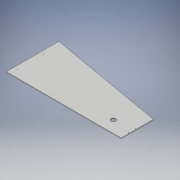
# Autodesk Inventor part: pinball-case-left-wall-outer
Saved by Autodesk Inventor 2017 (Build 210142000, 142)
## iProperties
Created: 2017-02-27
Part Number: pinball-case-left-wall-outer
Material: Generic
Document SubType Name: Modeling
Designer: John
Density: 1 g/cm^3
Appearance: Default
Author: John
Autodesk Inventor part; units mm, degrees
ref_plane "YZ Plane" through (0, 0, 0) normal (1, 0, 0) x (0, 1, 0)
ref_plane "XZ Plane" through (0, 0, 0) normal (0, 1, 0) x (-1, 0, 0)
ref_plane "XY Plane" through (0, 0, 0) normal (0, 0, 1) x (1, 0, 0)
sketch "Sketch1" plane through (0, 0, 0) normal (0, 1, 0) x (-1, 0, 0)
  line L0 (0, 0) -> (-590, 0)
  line L1 (-590, 0) -> (-590, -165.9671)
  line L2 (-590, -165.9671) -> (0, -165.9671)
  line L3 (0, -165.9671) -> (0, 0)
  line L4 (0, -165.9671) -> (0, -270)
  line L5 (0, -270) -> (-590, -165.9671)
  dimension "d0" = 590
  dimension "d28" = 270
  dimension "d29" = 10
  constraints: 12 end point, 2 parallel, 1 horizontal, 1 perpendicular, 1 vertical
  measures "d0" distance of L2.end L1.end
  measures "d28" distance of L0.start L4.end
  measures "d29" angle of L2 L5
extrude "Extrusion1" add sketch "Sketch1" along normal blind 3
sketch "Sketch3" plane through (0, 3, 0) normal (0, 1, 0) x (1, 0, 0)
  circle A0 centre (585.75, 41.75) radius 1.25
  circle A1 centre (585.75, 78.75) radius 1.25
  line L0 (590, 0) -> (590, 165.9671) projected
  line L1 (0, 0) -> (590, 0) projected
  dimension "d15" = 2.5
  dimension "d16" = 4.25
  dimension "d17" = 4.25
  dimension "d18" = 2.5
  dimension "d19" = 41.75
  dimension "d20" = 37
  constraints: 2 centre point
  measures "d15" diameter of A0
  measures "d16" distance from line of L0 A1.centre
  measures "d17" distance from line of L0 A0.centre
  measures "d18" diameter of A1
  measures "d19" distance from line of L1 A0.centre
  measures "d20" distance of A1.centre A0.centre
extrude "Extrusion3" cut sketch "Sketch3" along normal through all both and the other way through all
sketch "Sketch4" plane through (0, 3, 0) normal (0, 1, 0) x (1, 0, 0)
  circle A0 centre (490, 60) radius 12
  line L0 (0, 0) -> (590, 0) projected
  line L1 (590, 0) -> (590, 165.9671) projected
  line L2 (14.1705, 156) -> (20.1705, 156)
  line L3 (20.1705, 156) -> (20.1705, 144)
  line L4 (20.1705, 144) -> (14.1705, 144)
  line L5 (14.1705, 144) -> (14.1705, 156)
  line L6 (15, 114) -> (21, 114)
  line L7 (21, 114) -> (21, 102)
  line L8 (21, 102) -> (15, 102)
  line L9 (15, 102) -> (15, 114)
  line L10 (15, 72) -> (21, 72)
  line L11 (21, 72) -> (21, 60)
  line L12 (21, 60) -> (15, 60)
  line L13 (15, 60) -> (15, 72)
  circle A1 centre (17.1705, 176) radius 1.25
  circle A2 centre (18, 40) radius 1.25
  line L14 (18, 60) -> (18, 40) construction
  dimension "d23" = 24
  dimension "d24" = 60
  dimension "d25" = 100
  dimension "d30" = 6
  dimension "d31" = 12
  dimension "d32" = 30
  dimension "d33" = 30
  dimension "d34" = 2.5
  dimension "d35" = 2.5
  dimension "d36" = 20
  dimension "d37" = 20
  dimension "d38" = 60
  constraints: 26 end point, 9 parallel, 3 centre point, 3 horizontal, 3 perpendicular, 2 point on line, 1 midpoint, 1 vertical
  measures "d23" diameter of A0
  measures "d24" distance from line of L0 A0.centre
  measures "d25" distance from line of L1 A0.centre
  measures "d30" distance of L4.start L4.end
  measures "d31" distance of L3.start L4.start
  measures "d32" distance between parallel lines of L4 L6
  measures "d33" distance between parallel lines of L10 L8
  measures "d34" diameter of A1
  measures "d35" diameter of A2
  measures "d36" distance from line of L14.end L12
  measures "d37" distance from line of L2 A1.centre
  measures "d38" distance from line of L0 L14.start
extrude "Extrusion4" cut sketch "Sketch4" against normal through all contours A0 | A1 | A2
equation "\"d16\" = d17"
equation "\"d18\" = d15"
equation "\"d33\" = d32"
equation "\"d34\" = d35"
equation "\"d37\" = d36"
body "Solid1"
